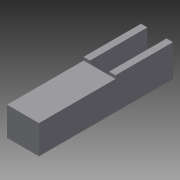
# Autodesk Inventor part: Limit Switch Container
Saved by Autodesk Inventor 2015 (Build 190159000, 159)
## iProperties
Created: 2015-01-22
Part Number: Limit Switch Container
Material: Generic
Document SubType Name: Modeling
Designer: nilesstanton
Density: 1 g/cm^3
Appearance: Default
Author: nilesstanton
Autodesk Inventor part; units mm, degrees
ref_plane "YZ Plane" through (0, 0, 0) normal (1, 0, 0) x (0, 1, 0)
ref_plane "XZ Plane" through (0, 0, 0) normal (0, 1, 0) x (-1, 0, 0)
ref_plane "XY Plane" through (0, 0, 0) normal (0, 0, 1) x (1, 0, 0)
sketch "Sketch1" plane through (0, 0, 0) normal (0, 1, 0) x (-1, 0, 0)
  line L0 (0, 0) -> (0, -28.575)
  line L1 (0, 0) -> (15.875, 0)
  line L2 (15.875, 0) -> (15.875, -28.575)
  line L3 (0, -28.575) -> (15.875, -28.575)
  dimension "d0" = 28.575
  dimension "d1" = 15.875
  constraints: 8 end point, 2 vertical, 1 horizontal, 1 perpendicular
  measures "d0" distance of L0.start L0.end
  measures "d1" distance of L0.start L1.end
extrude "Extrusion1" add sketch "Sketch1" along normal blind 22.225
sketch "Sketch2" plane through (-15.875, 0, 0) normal (0, 0, 1) x (1, 0, 0)
  line L0 (3.175, 3.175) -> (12.7, 3.175)
  line L1 (12.7, 3.175) -> (12.7, 19.05)
  line L2 (12.7, 19.05) -> (3.175, 19.05)
  line L3 (3.175, 19.05) -> (3.175, 3.175)
  line L4 (0, 0) -> (15.875, 0) construction
  line L5 (15.875, 0) -> (15.875, 22.225) construction
  line L6 (15.875, 22.225) -> (0, 22.225) construction
  line L7 (0, 22.225) -> (0, 0) construction
  dimension "d4" = 9.525
  dimension "d5" = 15.875
  dimension "d6" = 3.175
  dimension "d7" = 3.175
  dimension "d8" = 3.175
  constraints: 16 end point, 4 parallel, 2 horizontal, 2 perpendicular, 1 coincident
  measures "d4" distance of L0.start L0.end
  measures "d5" distance of L2.end L0.start
  measures "d6" distance between parallel lines of L3 L7
  measures "d7" distance between parallel lines of L5 L1
  measures "d8" distance between parallel lines of L6 L2
extrude "Extrusion2" cut sketch "Sketch2" against normal blind 50.8
sketch "Sketch3" plane through (-15.875, 0, 0) normal (0, 0, 1) x (1, 0, 0)
  line L0 (15.875, 0) -> (15.875, 22.225) projected
  line L1 (0, 22.225) -> (15.875, 22.225)
  line L2 (15.875, 22.225) -> (15.875, 19.05)
  line L3 (15.875, 19.05) -> (0, 19.05)
  line L4 (0, 19.05) -> (0, 22.225)
  line L5 (3.175, 19.05) -> (12.7, 19.05) construction
  line L6 (3.175, 19.05) -> (12.7, 19.05) projected
  constraints: 10 end point, 3 equal length, 2 point on line, 1 horizontal, 1 perpendicular
extrude "Extrusion3" cut sketch "Sketch3" against normal blind 50.8
sketch "Sketch4" plane through (-15.875, 0, 0) normal (0, 0, 1) x (1, 0, 0)
  line L0 (15.875, 0) -> (15.875, 19.05) projected
  line L1 (0, 0) -> (15.875, 0)
  line L2 (15.875, 0) -> (15.875, 3.175)
  line L3 (15.875, 3.175) -> (0, 3.175)
  line L4 (0, 3.175) -> (0, 0)
  point P0 (12.7, 3.175)
  constraints: 8 end point, 2 parallel, 2 point on line, 1 horizontal, 1 perpendicular
extrude "Extrusion4" cut sketch "Sketch4" against normal blind 50.8
sketch "Sketch5" plane through (-15.875, 19.05, 0) normal (0, 0, 1) x (1, 0, 0)
  line L0 (0, -15.875) -> (0, -1.5875)
  line L1 (0, -15.875) -> (3.175, -15.875)
  line L2 (0, -15.875) -> (3.175, -15.875) projected
  line L3 (3.175, -15.875) -> (3.175, -1.5875)
  line L4 (12.7, -15.875) -> (15.875, -15.875)
  line L5 (15.875, -15.875) -> (12.7, -15.875) projected
  line L6 (15.875, -15.875) -> (15.875, -1.5875)
  line L7 (12.7, -15.875) -> (12.7, -1.5875)
  line L8 (0, -1.5875) -> (3.175, -1.5875)
  line L9 (0, -15.875) -> (0, 0) projected
  line L10 (15.875, -1.5875) -> (12.7, -1.5875)
  line L11 (12.7, -15.875) -> (12.7, 0) projected
  line L12 (3.175, 0) -> (0, 0) projected
  line L13 (15.875, 0) -> (12.7, 0) projected
  line L14 (12.7, -15.875) -> (15.875, -15.875) projected
  line L15 (15.875, -15.875) -> (15.875, 0) projected
  point P0 (15.875, -19.05)
  dimension "d15" = 1.5875
  dimension "d16" = 1.5875
  dimension "d17" = 14.2875
  constraints: 16 end point, 6 perpendicular, 2 collinear, 1 parallel
  measures "d15" distance between parallel lines of L8 L12
  measures "d16" distance between parallel lines of L13 L10
  measures "d17" distance of L4.end L6.end
extrude "Extrusion5" add sketch "Sketch5" along normal blind 6.35 contours L0 L8 L3 L1 | L7 L10 L6 L4
sketch "Sketch6" plane through (-3.175, 19.05, -28.575) normal (-1, 0, 0) x (0, 0, 1)
  line L0 (34.925, -15.875) -> (0, -15.875) projected
  line L1 (34.925, -1.5875) -> (28.575, -1.5875)
  line L2 (28.575, -1.5875) -> (28.575, -15.875)
  line L3 (28.575, -15.875) -> (34.925, -15.875)
  line L4 (34.925, -15.875) -> (34.925, -1.5875)
  point P0 (28.575, -19.05)
  dimension "d20" = 6.35
  constraints: 8 end point, 2 parallel, 1 horizontal, 1 perpendicular, 1 point on line
  measures "d20" distance between parallel lines of L4 L2
extrude "Extrusion6" add sketch "Sketch6" along normal blind 9.525
sketch "Sketch7" plane through (-15.875, 19.05, 6.35) normal (0, 0, 1) x (1, 0, 0)
  line L0 (0, -15.875) -> (15.875, -15.875)
  line L1 (15.875, -15.875) -> (15.875, -1.5875)
  line L2 (15.875, -1.5875) -> (0, -1.5875)
  line L3 (0, -1.5875) -> (0, -15.875)
  point P0 (15.875, -19.05)
  constraints: 8 end point, 2 parallel, 1 horizontal, 1 perpendicular
extrude "Extrusion7" add sketch "Sketch7" along normal blind 31.75
body "Solid1"
